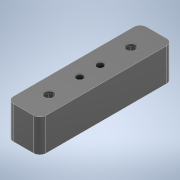
# Autodesk Inventor part: Base
Saved by Autodesk Inventor 2022 (Build 260153000, 153)
## iProperties
Created: 2021-11-22
Part Number: Base
Material: Genérico
Document SubType Name: Modeling
Designer: JK
Density: 1 g/cm^3
Appearance: Suave - Negro
Author: JK
Autodesk Inventor part; units mm, degrees
ref_plane "YZ Plane" through (0, 0, 0) normal (1, 0, 0) x (0, 1, 0)
ref_plane "XZ Plane" through (0, 0, 0) normal (0, 1, 0) x (-1, 0, 0)
ref_plane "XY Plane" through (0, 0, 0) normal (0, 0, 1) x (1, 0, 0)
sketch "Boceto1" plane through (0, 0, 0) normal (0, 1, 0) x (-1, 0, 0)
  line L0 (-8, 32.5) -> (8, 32.5)
  line L1 (8, 32.5) -> (8, -32.5)
  line L2 (8, -32.5) -> (-8, -32.5)
  line L3 (-8, -32.5) -> (-8, 32.5)
  line L4 (-8, 32.5) -> (8, -32.5) construction
  line L5 (8, 32.5) -> (-8, -32.5) construction
  line L6 (5.15, 26.15) -> (-5.15, 26.15)
  line L7 (-5.15, 26.15) -> (-5.15, 13.85)
  line L8 (-5.15, 13.85) -> (5.15, 13.85)
  line L9 (5.15, 13.85) -> (5.15, 26.15)
  line L10 (5.15, 26.15) -> (-5.15, 13.85) construction
  line L11 (-5.15, 26.15) -> (5.15, 13.85) construction
  line L12 (5.15, -13.85) -> (-5.15, -13.85)
  line L13 (-5.15, -13.85) -> (-5.15, -26.15)
  line L14 (-5.15, -26.15) -> (5.15, -26.15)
  line L15 (5.15, -26.15) -> (5.15, -13.85)
  line L16 (5.15, -13.85) -> (-5.15, -26.15) construction
  line L17 (-5.15, -13.85) -> (5.15, -26.15) construction
  point P0 (0, 0)
  point P1 (0, 20)
  point P2 (0, -20)
  point P3 (0, 20)
  point P4 (0, 0)
  point P5 (0, -20)
  point P6 (0, 0)
  dimension "d0" = 12.3
  dimension "d1" = 10.3
  dimension "d2" = 20
  dimension "d3" = 65
  dimension "d4" = 20
  dimension "d5" = 16
  constraints: 36 end point, 10 midpoint, 6 parallel, 3 horizontal, 3 perpendicular, 2 equal length, 2 vertical alignment
  measures "d0" distance of L8.end L6.start
  measures "d1" distance of L7.end L8.end
  measures "d2" distance of point (0, 0) point (0, 20)
  measures "d3" distance of L0.end L1.end
  measures "d4" distance of point (0, 0) point (0, -20)
  measures "d5" distance of L1.end L2.end
extrude "Extrusión1" add sketch "Boceto1" along normal blind 15
sketch "Boceto2" plane through (0, 15, 0) normal (0, 1, 0) x (1, 0, 0)
  line L0 (8, 32.5) -> (-8, 32.5) projected
  line L1 (-8, 32.5) -> (-8, -32.5) projected
  line L2 (-8, -32.5) -> (8, -32.5) projected
  line L3 (8, -32.5) -> (8, 32.5) projected
  line L4 (-5.15, -26.15) -> (-5.15, -13.85) projected
  line L5 (-5.15, -13.85) -> (5.15, -13.85) projected
  line L6 (5.15, -13.85) -> (5.15, -26.15) projected
  line L7 (5.15, -26.15) -> (-5.15, -26.15) projected
  line L8 (-5.15, 13.85) -> (-5.15, 26.15) projected
  line L9 (-5.15, 26.15) -> (5.15, 26.15) projected
  line L10 (5.15, 26.15) -> (5.15, 13.85) projected
  line L11 (5.15, 13.85) -> (-5.15, 13.85) projected
  point P0 (0, 0)
extrude "Extrusión2" add sketch "Boceto2" along normal blind 1 contours L3 L2 L1 L0 | L4 L5 L6 L7 | L8 L9 L10 L11
sketch "Boceto3" plane through (0, 0, 0) normal (0, -1, 0) x (1, 0, 0)
  circle A0 centre (0, 20) radius 2.15
  circle A1 centre (0, -20) radius 2.15
  line L0 (-5.15, 13.85) -> (5.15, 13.85) projected
  line L1 (5.15, -13.85) -> (-5.15, -13.85) projected
  line L2 (5.15, 13.85) -> (5.15, 26.15) projected
  point P0 (0, 0)
  dimension "d10" = 4.3
  dimension "d11" = 6.15
  dimension "d12" = 6.15
  dimension "d13" = 5.15
  constraints: 2 centre point, 1 equal radius, 1 vertical alignment
  measures "d10" diameter of A0
  measures "d11" distance from line of L0 A0.centre
  measures "d12" distance from line of L1 A1.centre
  measures "d13" distance from line of L2 A0.centre
extrude "Extrusión3" cut sketch "Boceto3" against normal through all
fillet "Empalme1" radius 1.15 8 edges at (5.15, 7.5, -13.85) (5.15, 7.5, 26.15) (5.15, 7.5, 13.85) (5.15, 7.5, -26.15) (-5.15, 7.5, -26.15) (-5.15, 7.5, 13.85) (-5.15, 7.5, -13.85) (-5.15, 7.5, 26.15)
fillet "Empalme2" radius 3 4 edges at (8, 8, -32.5) (8, 8, 32.5) (-8, 8, 32.5) (-8, 8, -32.5)
sketch "Boceto4" plane through (0, 16, 0) normal (0, 1, 0) x (1, 0, 0)
  circle A0 centre (0, -5) radius 1.7
  circle A1 centre (0, 5) radius 1.7
  point P0 (0, 0)
  dimension "d19" = 3.4
  dimension "d25" = 5
  dimension "d26" = 5
  constraints: 2 centre point, 1 equal radius
  measures "d19" diameter of A0
  measures "d25" distance of A1.centre point (0, 0)
  measures "d26" distance of point (0, 0) A0.centre
extrude "Extrusión4" cut sketch "Boceto4" against normal through all
sketch "Boceto5" plane through (0, 0, 0) normal (0, -1, 0) x (1, 0, 0)
  circle A0 centre (0, 5) radius 1.7 projected
  circle A1 centre (0, 5) radius 2.8
  circle A2 centre (0, -5) radius 1.7 projected
  circle A3 centre (0, -5) radius 2.8
  line L0 (3.2332, 5) -> (1.6166, 2.2)
  line L1 (1.6166, 2.2) -> (-1.6166, 2.2)
  line L2 (-1.6166, 2.2) -> (-3.2332, 5)
  line L3 (-3.2332, 5) -> (-1.6166, 7.8)
  line L4 (-1.6166, 7.8) -> (1.6166, 7.8)
  line L5 (1.6166, 7.8) -> (3.2332, 5)
  line L6 (3.2332, -5) -> (1.6166, -7.8)
  line L7 (1.6166, -7.8) -> (-1.6166, -7.8)
  line L8 (-1.6166, -7.8) -> (-3.2332, -5)
  line L9 (-3.2332, -5) -> (-1.6166, -2.2)
  line L10 (-1.6166, -2.2) -> (1.6166, -2.2)
  line L11 (1.6166, -2.2) -> (3.2332, -5)
  point P0 (0, 0)
  dimension "d27" = 5.6
  constraints: 24 end point, 4 coincident, 2 centre point, 2 horizontal alignment, 2 tangent, 1 equal radius, 26 other
  measures "d27" diameter of A1
extrude "Extrusión5" cut sketch "Boceto5" against normal blind 5 contours A0 | A1 | A1 L5 L0 | A1 L4 L5 | L0 L1 A1 | A1 L3 L4 | L1 L2 A1 | A1 L2 L3 | A2 | A3 | A3 L11 L6 | A3 L10 L11 | L6 L7 A3 | A3 L9 L10 | L7 L8 A3 | A3 L8 L9
equation "\"d4\" = d2"
